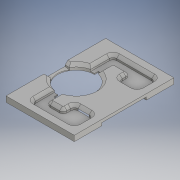
# Autodesk Inventor part: wide_access_platform_v01
Saved by Autodesk Inventor 2016 (Build 200138000, 138)
## iProperties
Company: HMS
Created: 2016-07-11
Part Number: wide_access_platform_v01
Material: Generic
Document SubType Name: Modeling
Designer: Stephen Holtz
Density: 1 g/cm^3
Appearance: Default
Author: Stephen Holtz
Title: Wide Access Drosophila Physiology Platform
Autodesk Inventor part; units mm, degrees
ref_plane "YZ Plane" through (0, 0, 0) normal (1, 0, 0) x (0, 1, 0)
sketch "Base" plane through (0, 0, 0) normal (0, 1, 0) x (-1, 0, 0)
  line L0 (18, 27) -> (18, -27)
  line L1 (18, -27) -> (-18, -27)
  line L2 (-18, -27) -> (-18, 27)
  line L3 (-18, 27) -> (18, 27)
  line L4 (18, 27) -> (-18, -27) construction
  line L5 (18, -27) -> (-18, 27) construction
  line L6 (8, 27) -> (8, -27) construction
  circle A0 centre (8, 0) radius 10
  line L7 (18, 27) -> (19, 27)
  line L8 (19, 27) -> (19, -27)
  line L9 (19, -27) -> (18, -27)
  line L10 (18, -27) -> (18, 27)
  point P0 (0, 0)
  dimension "d10" = 54
  dimension "d12" = 20
  dimension "d78" = 26
  dimension "d79" = 1
  constraints: 22 end point, 4 parallel, 3 midpoint, 3 perpendicular, 2 point on line, 1 centre point, 1 collinear, 1 horizontal, 1 tangent, 1 vertical
  measures "d10" distance of L1.end L2.end
  measures "d12" diameter of A0
  measures "d78" distance from line of L2 A0.centre
  measures "d79" distance of L8.end L9.end
extrude "Extrusion7" add sketch "Base" along normal blind 3
sketch "Mid Profile" plane through (0, 0, 0) normal (0, 0, 1) x (1, 0, 0)
  line L0 (18, 0) -> (-18, 0) construction
  line L1 (-18, 0) -> (-19, 0) projected
  line L2 (-8, 0) -> (-9, 0)
  line L3 (-8, 0) -> (18, 0)
  line L4 (18, 0) -> (18, 1.5)
  line L5 (18, 1.5) -> (-8, 1.5)
  line L6 (-8, 1.5) -> (-8, 0)
  line L7 (18, 0) -> (18, 3) projected
  line L8 (-19, 3) -> (18, 3) projected
  line L9 (-9, 0) -> (-8, 1.5)
  point P0 (0, 0)
  point P1 (-8, 0)
  point P2 (-18, 0)
  point P3 (-19, 0)
  dimension "d92" = 1
  dimension "d93" = 1.5
  constraints: 12 end point, 2 parallel, 1 collinear, 1 horizontal, 1 perpendicular, 2 other
  measures "d92" distance of L2.start L2.end
  measures "d93" distance between parallel lines of L5 L8
sketch "Bath" plane through (0, 3, 0) normal (0, 1, 0) x (1, 0, 0)
  circle A0 centre (-8, 0) radius 10 construction
  line L0 (-19, -27) -> (18, -27) construction
  line L1 (-19, 27) -> (-19, -27) construction
  line L2 (18, 27) -> (-19, 27) construction
  line L3 (18, -27) -> (18, 27) construction
  line L4 (-8, -27) -> (-8, 27) construction
  line L5 (-10, 0) -> (-10, 20)
  line L6 (-10, 22) -> (-6, 22)
  line L7 (-6, 16) -> (-6, 0)
  line L8 (-6, 0) -> (-10, 0)
  line L9 (-19, 27) -> (-19, -27) projected
  line L10 (-19, 0) -> (18, 0)
  line L11 (-10, 0) -> (-8, 0) construction
  line L12 (-8, 22) -> (11, 22)
  line L13 (13, 22) -> (13, 18) construction
  line L14 (13, 18) -> (-10, 18) construction
  line L15 (-10, 18) -> (-10, 22) construction
  line L16 (13, 22) -> (3, 22)
  line L17 (3, 16) -> (3, 14)
  line L18 (5, 12) -> (11, 12)
  line L19 (13, 14) -> (13, 20)
  line L20 (1, 18) -> (-4, 18)
  arc A1 (-8, 22) -> (-10, 20) centre (-8, 20) ccw
  arc A2 (-4, 18) -> (-6, 16) centre (-4, 16) ccw
  arc A3 (3, 16) -> (1, 18) centre (1, 16) ccw
  arc A4 (13, 20) -> (11, 22) centre (11, 20) ccw
  arc A5 (11, 12) -> (13, 14) centre (11, 14) ccw
  arc A6 (3, 14) -> (5, 12) centre (5, 14) ccw
  line L21 (-10, 0) -> (-10, -20)
  line L22 (-6, -16) -> (-6, 0)
  line L23 (-8, -22) -> (11, -22)
  line L24 (3, -16) -> (3, -14)
  line L25 (5, -12) -> (11, -12)
  line L26 (13, -14) -> (13, -20)
  line L27 (1, -18) -> (-4, -18)
  arc A7 (-10, -20) -> (-8, -22) centre (-8, -20) ccw
  arc A8 (-6, -16) -> (-4, -18) centre (-4, -16) ccw
  arc A9 (1, -18) -> (3, -16) centre (1, -16) ccw
  arc A10 (11, -22) -> (13, -20) centre (11, -20) ccw
  arc A11 (13, -14) -> (11, -12) centre (11, -14) ccw
  arc A12 (5, -12) -> (3, -14) centre (5, -14) ccw
  line L28 (-19, -10) -> (18, -10)
  circle A13 centre (-8, 0) radius 10 projected
  point P0 (0, 0)
  point P1 (-8, 0)
  point P2 (13, 12)
  point P3 (3, 18)
  point P4 (-6, 18)
  dimension "d83" = 5
  dimension "channel_w" = 4
  dimension "d85" = 2
  dimension "d86" = 4
  dimension "d88" = 5
  dimension "d89" = 10
  dimension "d90" = 10
  dimension "d91" = 2
  constraints: 48 end point, 24 point on circle, 19 point on line, 18 symmetric about line, 13 tangent, 12 centre point, 6 parallel, 5 equal radius, 5 perpendicular, 4 midpoint, 2 horizontal, 1 coincident, 1 collinear, 1 vertical, 6 other
  measures "d83" distance between parallel lines of L2 L6
  measures "channel_w" distance between parallel lines of L7 L5
  measures "d85" distance of L5.start L11.end
  measures "d86" distance of L13.start L13.end
  measures "d88" distance between parallel lines of L3 L13
  measures "d89" distance of point (13, 12) L13.start
  measures "d90" distance between parallel lines of L19 L17
  measures "d91" radius of A1
ref_plane "Work Plane4" through (5, 3, 12) normal (0, 0, 1) x (1, 0, 0)
extrude "Extrusion8" cut sketch "Mid Profile" along normal up to surface (12 mm away) contours L6 L5 L4 L3
mirror "Mirror1" about plane through (0, 0, 0) normal (0, 0, 1) of "Extrusion8"
extrude "Extrusion9" cut sketch "Bath" against normal blind 2.5 contours L8 L22 A13 L21 | A13 L28 L21 | L22 L28 A13 | L28 L22 A8 L27 A9 L24 A12 L25 A11 L26 A10 L23 A7 L21
chamfer "Chamfer6" distance 1.5 angle 45 13 edges at (-1.5, 3, 18) (2.4142, 3, 17.4142) (3, 3, 15) (3.5858, 3, 12.5858) (8, 3, 12) (12.4142, 3, 12.5858) (13, 3, 17) (12.4142, 3, 21.4142) (1.5, 3, 22) (-9.4142, 3, 21.4142) (-10, 3, 14.899) (-5.4142, 3, 17.4142) (-6, 3, 12.899)
mirror "Mirror2" about plane through (0, 0, 0) normal (0, 0, 1) of "Extrusion9", "Chamfer6"
chamfer "Chamfer7" distance 1.5 angle 45 1 edges at (2, 3, 0)
chamfer "Chamfer8" distance 1.5 angle 45 1 edges at (-18, 3, 0)
sketch "Sketch14" plane through (0, 0, 0) normal (0, 0, 1) x (1, 0, 0)
  line L0 (-19.5492, 0) -> (-19.5492, 5.1244)
  line L1 (-19.5492, 1) -> (-13.2592, -0.6854)
  line L2 (-13.2592, -0.6854) -> (-13.2592, 5.1244)
  line L3 (-11.5, 5.1244) -> (-19.5492, 5.1244)
  line L4 (-19.5492, 5.1244) -> (-19.5492, 1)
  line L5 (-13.2592, 5.1244) -> (-19.5492, 5.1244)
  line L6 (18, 3) -> (-19.5492, 3) projected
  line L7 (18, 0) -> (-19.5492, 0) projected
  point P0 (0, 0)
  dimension "d125" = 1
  dimension "d126" = 75
  constraints: 12 end point, 2 point on line, 1 other
  measures "d125" distance from line of L7 L1.start
  measures "d126" angle of L1 L2
extrude "Extrusion11" cut sketch "Sketch14" along normal mid plane 10 contours L0 L6 L2 L7 L1 | L7 L2 L1 | L0 L3 L2 L6
chamfer "Chamfer10" distance 1.5 angle 45 1 edges at (-18.6781, 3, -5)
chamfer "Chamfer11" distance 1.5 angle 45 1 edges at (-18.6781, 3, 5)
ref_plane "Work Plane5" through (-6.75, 3, -10.5) normal (0, 0, 1) x (1, 0, 0)
equation "\"d85\" = 0.5 * channel_w"
equation "\"d86\" = channel_w"
equation "\"d89\" = 2.5 * channel_w"
equation "\"d90\" = 2.5 * channel_w"
body "Solid4"
